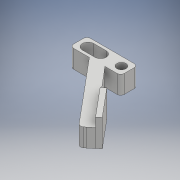
# Autodesk Inventor part: finger_3
Saved by Autodesk Inventor 2018 (Build 220112000, 112)
## iProperties
Created: 2019-01-21
Part Number: finger_3
Material: 一般
Document SubType Name: Modeling
Designer: lowyu
Density: 1 g/cm^3
Appearance: 既定
Mass: 4.12708 g
Surface Area: 29.3516 cm^2
Volume: 4.12708 cm^3
Author: lowyu
Autodesk Inventor part; units mm, degrees
ref_plane "YZ Plane" through (0, 0, 0) normal (1, 0, 0) x (0, 1, 0)
ref_plane "XZ Plane" through (0, 0, 0) normal (0, 1, 0) x (-1, 0, 0)
ref_plane "XY Plane" through (0, 0, 0) normal (0, 0, 1) x (1, 0, 0)
sketch "スケッチ1" plane through (0, 0, 0) normal (0, 0, 1) x (1, 0, 0)
  line L0 (18.408, 0) -> (-1.0303, 0)
  arc A0 (36.165, -44.7764) -> (37.2594, -44.8743) centre (37.0041, -41.5628) ccw
  line L1 (38.972, -43.427) -> (37.2594, -44.8743)
  line L2 (31.483, -28.9072) -> (15.1835, -9.4196)
  circle A1 centre (19.5337, -4.7196) radius 2.5
  line L3 (8.0337, -1.575) -> (1.1379, -1.575)
  arc A2 (7.8277, -7.8182) -> (8.0337, -1.575) centre (8.0337, -4.7) ccw
  line L4 (7.8277, -7.8182) -> (1.0695, -7.8243)
  arc A3 (1.1379, -1.575) -> (1.0695, -7.8243) centre (1.1379, -4.7) ccw
  line L5 (36.165, -44.7764) -> (6.576, -9.4)
  line L6 (18.408, 0) -> (23.7968, 0)
  line L7 (23.7968, 0) -> (23.7968, -8.35)
  line L8 (-1.0303, 0) -> (-4.1421, 0)
  line L9 (-4.1421, 0) -> (-4.1421, -7.7348)
  line L10 (-4.1421, -7.7348) -> (-4.1421, -9.4)
  line L11 (-4.1421, -9.4) -> (6.576, -9.4)
  line L12 (15.1835, -9.4196) -> (23.7968, -9.4196)
  line L13 (23.7968, -9.4196) -> (23.7968, -7.7545)
  line L14 (41.7112, -41.1359) -> (41.7109, -41.1356)
  line L15 (41.7109, -41.1356) -> (43.7109, -39.4628)
  line L16 (43.7109, -39.4628) -> (30.8794, -24.1216)
  line L17 (30.8794, -24.1216) -> (28.8794, -25.7944)
  line L18 (38.972, -43.427) -> (41.7112, -41.1359)
  line L19 (31.483, -28.9072) -> (41.7112, -41.1359)
  point P0 (0, 0)
  point P1 (0, 0)
  dimension "d0" = 5
  dimension "d1" = 3.125
  dimension "d3" = 11.5
  dimension "d5" = 4.7
  dimension "d9" = 3.125
  dimension "d11" = 4.7
  dimension "d12" = 4.7
  dimension "d13" = 6.8958
  dimension "d14" = 20
  dimension "d19" = 2
  dimension "d24" = 46.1194
  dimension "d25" = 41.3474
  constraints: 41 end point, 6 perpendicular, 6 point on circle, 4 centre point, 3 point on line, 2 horizontal, 2 parallel, 1 coincident, 1 collinear, 1 vertical
  measures "d0" diameter of A1
  measures "d1" radius of A2
  measures "d3" distance of point (19.534, -4.72) A2.centre
  measures "d5" distance from line of L0 A3.centre
  measures "d9" radius of A3
  measures "d11" distance from line of L11 A3.centre
  measures "d12" distance from line of point (19.534, -4.72) L12
  measures "d13" distance of A2.centre A3.centre
  measures "d14" distance of L15.end L16.end
  measures "d19" horizontal distance of L16.end L17.end
  measures "d24" distance of L5.start L5.end
  measures "d25" distance from line of L2.end L15
extrude "押し出し1" add sketch "スケッチ1" along normal blind 10
fillet "フィレット1" radius 2 4 edges at (23.7968, 0, 5) (23.7968, -9.4196, 5) (-4.1421, 0, 5) (-4.1421, -9.4, 5)
fillet "フィレット2" radius 2 2 edges at (37.2594, -44.8743, 5) (36.165, -44.7764, 5)
sketch "スケッチ4" plane through (0, 0, 10) normal (0, 0, 1) x (1, 0, 0)
  line L0 (30.8794, -24.1216) -> (28.8794, -25.7944) projected
  line L1 (43.7109, -39.4628) -> (30.8794, -24.1216) projected
  line L2 (41.7109, -41.1356) -> (43.7109, -39.4628) projected
  line L3 (28.8794, -25.7944) -> (41.7109, -41.1356)
  line L4 (43.7109, -39.4628) -> (41.7109, -41.1356)
  line L5 (28.8794, -25.7944) -> (30.8794, -24.1216)
  line L6 (30.8794, -24.1216) -> (43.7109, -39.4628)
  point P0 (0, 0)
  constraints: 8 end point, 1 collinear
extrude "押し出し4" add sketch "スケッチ4" along normal blind 5
equation "\"d5\" = d11"
equation "\"d9\" = d1"
